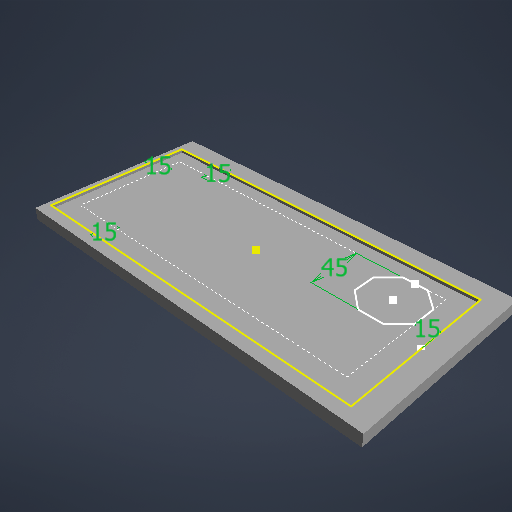
# Autodesk Inventor part: tray_multipart
Saved by Autodesk Inventor 2026 (Build 300175050, 175E)
## iProperties
Part Number: tray_multipart
Material: Generic
Document SubType Name: Modeling
Designer: romanov
Appearance: Default
Author: romanov
Autodesk Inventor part; units mm, degrees
ref_plane "YZ Plane" through (0, 0, 0) normal (1, 0, 0) x (0, 1, 0)
ref_plane "XZ Plane" through (0, 0, 0) normal (0, 1, 0) x (-1, 0, 0)
ref_plane "XY Plane" through (0, 0, 0) normal (0, 0, 1) x (1, 0, 0)
sketch "Sketch1" plane through (0, 0, 0) normal (0, 1, 0) x (-1, 0, 0)
  line L0 (150, 75) -> (-150, 75)
  line L1 (-150, 75) -> (-150, -75)
  line L2 (-150, -75) -> (150, -75)
  line L3 (150, -75) -> (150, 75)
  line L4 (150, 75) -> (-150, -75) construction
  line L5 (-150, 75) -> (150, -75) construction
  point P0 (0, 0)
  dimension "d0" = 300
  dimension "d1" = 150
  constraints: 12 end point, 2 midpoint, 2 parallel, 1 horizontal, 1 perpendicular
  measures "d0" distance between parallel lines of L1 L3
  measures "d1" distance between parallel lines of L0 L2
extrude "Extrusion1" add sketch "Sketch1" along normal blind 10
sketch "Sketch3" plane through (0, 10, 0) normal (0, 1, 0) x (1, 0, 0)
  line L0 (-145, -65) -> (134, -65)
  line L1 (134, -65) -> (134, 59)
  line L2 (134, 59) -> (-145, 59)
  line L3 (-145, 59) -> (-145, -65)
  line L4 (-150, 75) -> (-150, -75) projected
  line L5 (-150, -75) -> (150, -75) projected
  point P0 (0, 0)
  dimension "d4" = 279
  dimension "d5" = 124
  dimension "d6" = 5
  dimension "d7" = 10
  constraints: 8 end point, 2 parallel, 1 horizontal, 1 perpendicular
  measures "d4" distance of L1.end L2.end
  measures "d5" distance of L0.end L1.end
  measures "d6" distance between parallel lines of L4 L3
  measures "d7" distance between parallel lines of L5 L0
extrude "Extrusion2" cut sketch "Sketch3" against normal blind 3
sketch "Sketch4" plane through (0, 10, 0) normal (0, 1, 0) x (1, 0, 0)
  line L0 (-130, 44) -> (119, 44) construction
  line L1 (119, 44) -> (119, -50) construction
  line L2 (119, -50) -> (-130, -50) construction
  line L3 (-130, -50) -> (-130, 44) construction
  line L4 (-145, 59) -> (134, 59) projected
  line L5 (-145, -65) -> (-145, 59) projected
  line L6 (134, -65) -> (-145, -65) projected
  line L7 (134, 59) -> (134, -65) projected
  line L8 (105.8198, 44) -> (119, 30.8198)
  line L9 (119, 30.8198) -> (119, 12.1802)
  line L10 (119, 12.1802) -> (105.8198, -1)
  line L11 (105.8198, -1) -> (87.1802, -1)
  line L12 (87.1802, -1) -> (74, 12.1802)
  line L13 (74, 12.1802) -> (74, 30.8198)
  line L14 (74, 30.8198) -> (87.1802, 44)
  line L15 (87.1802, 44) -> (105.8198, 44)
  point P0 (0, 0)
  point P1 (134, -3)
  point P2 (96.5, 21.5)
  point P3 (96.5, 44)
  dimension "d10" = 15
  dimension "d11" = 15
  dimension "d12" = 15
  dimension "d13" = 15
  dimension "d14" = 45
  constraints: 24 end point, 2 collinear, 2 midpoint, 2 parallel, 1 horizontal, 1 perpendicular, 1 point on line, 17 other
  measures "d10" distance between parallel lines of L4 L0
  measures "d11" distance between parallel lines of L5 L3
  measures "d12" distance between parallel lines of L6 L2
  measures "d13" distance from line of point (134, -3) L1
  measures "d14" distance between parallel lines of L11 L0
equation "\"d4\" = pebble_width"
equation "\"d5\" = pebble_height"
equation "\"pebble_height\" = 124"
equation "\"pebble_width\" = 279"
equation "\"pebble_depth\" = 16"
body "Solid1"
